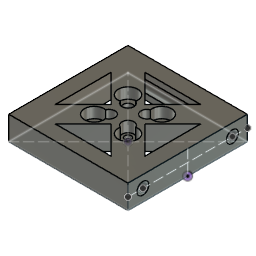
plate (Autodesk Fusion 360 design; units mm, degrees)
Autodesk Fusion 360 part; units mm, degrees
note: some values were not read from the file. Set by a fixed rule: the direction of a hole.
sketch "Sketch1" plane through (0, 0, 0) normal (0, 0, 1) x (1, 0, 0)
  line L0 (20, -20) -> (-20, -20)
  line L1 (-20, -20) -> (-20, 20)
  line L2 (-20, 20) -> (20, 20)
  line L3 (20, 20) -> (20, -20)
  line L4 (20, -20) -> (-20, 20) construction
  line L5 (-20, -20) -> (20, 20) construction
  dimension "d1" = 40
  dimension "d2" = 40
  constraint horizontal L0
  constraint perpendicular L0 L1
  constraint parallel L0 L2
  constraint parallel L1 L3
  constraint coincident L4 origin
  constraint coincident L5 origin
  measures "d1" distance of L1.end L2.end
  measures "d2" distance of L0.end L1.end
extrude "Extrude1" add sketch "Sketch1" along normal blind 8
sketch "Sketch2" plane through (20, 0, 0) normal (1, 0, 0) x (0, 1, 0)
  line L0 (-20, 0) -> (20, 0)
  line L1 (20, 0) -> (20, 8)
  line L2 (20, 8) -> (-20, 8)
  line L3 (-20, 8) -> (-20, 0)
  line L4 (-20, 4) -> (20, 4) construction
  line L5 (0, 8) -> (0, 0) construction
  point P0 (-15, 4)
  point P1 (15, 4)
  point P2 (-20, 4)
  point P3 (20, 4)
  dimension "d5" = 30
  constraint coincident L3 P2
  constraint midpoint L1 P3
  constraint midpoint L3 P2
  constraint coincident P2 L4.start
  constraint coincident P3 L4.end
  constraint coincident P0 L4
  constraint coincident P1 L4
  constraint midpoint L2 L5.start
  constraint coincident L5.end origin
  constraint symmetric P0 P1 L5
  measures "d5" distance of P0 P1
sketch "Sketch3" plane through (0, 0, 8) normal (0, 0, 1) x (-1, 0, 0)
  line L0 (-20, -20) -> (20, -20)
  line L1 (20, -20) -> (20, 20)
  line L2 (20, 20) -> (-20, 20)
  line L3 (-20, 20) -> (-20, -20)
  line L4 (-20, -20) -> (-20, 20)
  line L5 (-20, 20) -> (20, 20)
  line L6 (20, -20) -> (-20, -20)
  line L7 (20, 20) -> (20, -20)
  line L8 (-15, 15) -> (-15, -15)
  line L9 (-15, -15) -> (15, -15)
  line L10 (15, -15) -> (15, 15)
  line L11 (15, 15) -> (-15, 15)
  line L12 (15, 15) -> (-15, -15) construction
  line L13 (-15, 15) -> (15, -15) construction
  line L14 (9.3431, -15) -> (-15, 9.3431)
  line L15 (15, -9.3431) -> (-9.3431, 15)
  line L16 (9.3431, 15) -> (-15, -9.3431)
  line L17 (-9.3431, -15) -> (15, 9.3431)
  point P0 (5.6569, -5.6569)
  point P1 (-5.6569, 5.6569)
  point P2 (-5.6569, -5.6569)
  point P3 (5.6569, 5.6569)
  point P4 (3.182, 3.182)
  point P5 (-3.182, 3.182)
  point P6 (-3.182, -3.182)
  point P7 (3.182, -3.182)
  dimension "d24" = -5
  dimension "d25" = 8
  dimension "d26" = 8
  dimension "d49" = 16
  dimension "d50" = 9
  constraint coincident L9 L14.start
  constraint coincident L8 L14.end
  constraint coincident L10 L15.start
  constraint coincident L11 L15.end
  constraint parallel L14 L15
  constraint coincident L11 L16.start
  constraint coincident L8 L16.end
  constraint coincident L9 L17.start
  constraint coincident L10 L17.end
  constraint parallel L16 L17
  constraint symmetric L13 L14 L15
  constraint symmetric L12 L16 L17
  constraint coincident L13 P0
  constraint coincident L13 P1
  constraint coincident L12 P2
  constraint coincident L12 P3
  constraint horizontal P1 P3
  constraint vertical P0 P3
  constraint horizontal P0 P2
  constraint coincident L12 P4
  constraint coincident L13 P5
  constraint coincident L12 P6
  constraint coincident L13 P7
  constraint horizontal P4 P5
  constraint vertical P4 P7
  constraint horizontal P6 P7
  measures "d25" distance of L16 L17
  measures "d26" distance of L14 L15
  measures "d49" distance of P0 P1
  measures "d50" distance of P5 P7
extrude "Extrude3" cut sketch "Sketch3" against normal up to surface (8 mm away) contours L8 L14 L16 | L11 L15 L16 | L9 L14 L17 | L10 L15 L17
hole "Hole2" at (20, -15, 4) at (20, 15, 4) direction (-1, 0, 0) diameter 4 end up to surface (40 mm away)
hole "Hole3" at (-5.6569, 5.6569, 8) at (5.6569, 5.6569, 8) at (5.6569, -5.6569, 8) at (-5.6569, -5.6569, 8) direction (0, 0, -1) diameter 3.2 end up to surface (8 mm away) counterbore diameter 6.5 counterbore depth 3.6
hole "Hole4" at (-3.182, 3.182, 8) at (3.182, 3.182, 8) at (3.182, -3.182, 8) at (-3.182, -3.182, 8) direction (0, 0, -1) diameter 2.2 end up to surface (8 mm away) counterbore diameter 4 counterbore depth 3.6
sketch "Sketch5" plane through (0, 0, 0) normal (0, 0, 1) x (1, 0, 0)
hole "Hole6" at (0, 0, 0) direction (0, 0, 1) diameter 8 depth 3 tip angle 118
equation "d26 = d25"
